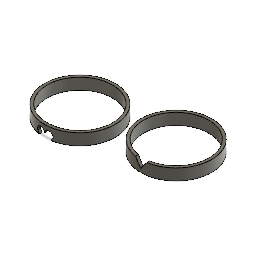
hringir v1 (Autodesk Fusion 360 design; units mm, degrees)
Autodesk Fusion 360 part; units mm, degrees
sketch "Sketch1" plane through (0, 0, 0) normal (0, 1, 0) x (1, 0, 0)
  circle A0 centre (0, 0) radius 8.5
  circle A1 centre (0, 0) radius 9.25
  dimension "d1" = 17
  dimension "d2" = 18.5
  constraint coincident A0.centre A1.centre
  measures "d1" diameter of A0
  measures "d2" diameter of A1
extrude "Extrude1" add sketch "Sketch1" along normal blind 3 makes body 1
extrude "Extrude2" add 1 faces at (8.9339, 3, 0.8818) along direction (0, 1, 0) blind 3 separate body on bodies 1 makes body 2
sketch "Sketch2" plane through (0, 0, 0) normal (0, 0, 1) x (1, 0, 0)
  line L0 (-1.908, 3.6971) -> (0, 1)
  line L1 (0, 1) -> (1.908, 3.6971)
  arc A0 (0, 4) -> (-1.9996, 3.9718) centre (-1, 4) ccw
  arc A1 (1.9996, 3.9718) -> (0, 4) centre (1, 4) ccw
  arc A2 (-1.9996, 3.9718) -> (-1.908, 3.6971) centre (-1.4998, 3.9859) ccw
  arc A3 (1.908, 3.6971) -> (1.9996, 3.9718) centre (1.4998, 3.9859) ccw
  dimension "d7" = 2
  dimension "d8" = 2
  dimension "d9" = 0.5
  dimension "d10" = 0.5
  constraint tangent A0 A2
  constraint tangent L0 A2
  constraint tangent L1 A3
  constraint tangent A1 A3
  measures "d7" diameter of A0
  measures "d8" diameter of A1
  measures "d9" radius of A2
  measures "d10" radius of A3
extrude "Extrude3" cut sketch "Sketch2" along normal through all bodies 1 2
move_body "Move1" bodies 2 to x (1, 0, 0) y (0, 1, 0) z (0, 0, 1) at (-20.4877, -3, 4.6102)
